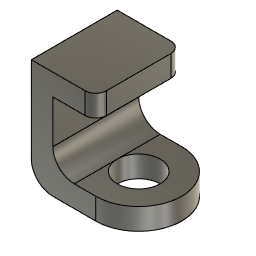
e3 (Autodesk Fusion 360 design; units mm, degrees)
Autodesk Fusion 360 part; units mm, degrees
sketch "Sketch1" plane through (0, 0, 0) normal (0, 0, 1) x (1, 0, 0)
  line L0 (0, 0) -> (20, 0)
  line L1 (20, 40) -> (0, 40)
  line L2 (0, 40) -> (0, 0)
  circle A0 centre (20, 20) radius 10
  arc A1 (20, 0) -> (20, 40) centre (20, 20) ccw
  dimension "d1" = 20
  dimension "d2" = 40
  dimension "d3" = 20
  dimension "d10" = 20
  constraint horizontal L0
  constraint horizontal L1
  constraint vertical L2
  constraint coincident L0.start L2.end
  constraint tangent L0 A1
  constraint concentric A0 A1
  measures "d1" distance of L0.start L0.end
  measures "d2" distance of L0.start L1.end
  measures "d3" diameter of A0
  measures "d10" radius of A1
sketch "Sketch2" plane through (0, 0, 0) normal (1, 0, 0) x (0, 1, 0)
  line L0 (0, 0) -> (40, 0)
  line L1 (40, 0) -> (40, 50.06)
  line L2 (40, 50.06) -> (0, 50.06)
  line L3 (0, 50.06) -> (0, 0)
  dimension "d4" = 40
  dimension "d5" = 50.06
  constraint horizontal L0
  constraint vertical L1
  constraint horizontal L2
  constraint vertical L3
  constraint coincident L0.start L3.end
  measures "d4" distance of L0.start L0.end
  measures "d5" distance of L0.start L2.end
ref_plane "WorkPlane1" through (20, 20, 50.06) normal (0, 0, 1) x (1, 0, 0)
sketch "Sketch3" plane through (20, 20, 50.06) normal (0, 0, 1) x (1, 0, 0)
  line L0 (-20, 20) -> (-5, 20)
  line L1 (0, 15) -> (0, -15)
  line L2 (-5, -20) -> (-20, -20)
  line L3 (-20, -20) -> (-20, 20)
  arc A0 (-5, -20) -> (0, -15) centre (-5, -15) ccw
  arc A1 (0, 15) -> (-5, 20) centre (-5, 15) ccw
  point P0 (0, 20)
  dimension "d7" = 20
  dimension "d8" = 40
  dimension "d9" = 5
  constraint horizontal L0
  constraint vertical L1
  constraint horizontal L2
  constraint vertical L3
  constraint tangent L2 A0
  constraint tangent L1 A0
  constraint coincident P0 L1
  constraint coincident P0 L0
  constraint tangent L1 A1
  constraint tangent L0 A1
  constraint equal A0 A1
  measures "d7" distance of L0.start P0
  measures "d8" distance of L0.start L2.end
  measures "d9" radius of A0
extrude "Extrude1" add sketch "Sketch1" along normal blind 10
extrude "Extrude2" add sketch "Sketch2" against normal blind 10
extrude "Extrude3" add sketch "Sketch3" against normal blind 10
fillet "Fillet1" radius 10 1 edges at (0, 20, 10)
fillet "Fillet2" radius 10 1 edges at (-10, 20, 0)
